Top_floor_v1 (Autodesk Fusion 360 design; units mm, degrees)
Autodesk Fusion 360 part; units mm, degrees
note: some values were not read from the file. Set by a fixed rule: which sketch regions a step uses.
other "Esquisse1"
sketch "Esquisse1" plane through (0, 0, 0) normal (0, 0, 1) x (1, 0, 0) in component "Component"
  line L0 (159, 101.837) -> (-151, 101.837)
  arc A0 (-151, 101.837) -> (-156, 96.837) centre (-151, 96.837) ccw
  line L1 (-156, 96.837) -> (-156, -18.163)
  line L2 (164, -123.163) -> (164, 96.837)
  arc A1 (164, 96.837) -> (159, 101.837) centre (159, 96.837) ccw
  arc A2 (159, -128.163) -> (164, -123.163) centre (159, -123.163) ccw
  line L3 (-26, -128.163) -> (159, -128.163)
  circle A3 centre (155, 92.837) radius 2.75
  circle A4 centre (-147, 92.837) radius 2.75
  circle A5 centre (155, -119.163) radius 2.75
  line L4 (-26, -128.163) -> (-151, -128.163)
  line L5 (-156, -123.163) -> (-156, -18.163)
  arc A6 (-156, -123.163) -> (-151, -128.163) centre (-151, -123.163) ccw
  circle A7 centre (-147, -119.163) radius 2.75
  point P0 (155, 92.837)
  point P1 (-147, 92.837)
  point P2 (155, -119.163)
  dimension "d5" = 5
  dimension "d6" = 5
  dimension "d7" = 5.5
  dimension "d8" = 5.5
  dimension "d9" = 9
  dimension "d10" = 9
  dimension "d11" = 9
  dimension "d12" = 9
  constraint coincident L3.start L4.start
  constraint perpendicular L1 L4
  constraint coincident L1.end L5.end
  constraint perpendicular L3 L5
  constraint tangent L4 A6
  constraint tangent L5 A6
  measures "d5" radius of A6
  measures "d6" radius of A2
  measures "d7" diameter of A7
  measures "d8" diameter of A3
  measures "d9" distance of L2 P0
  measures "d10" distance of L0 P0
  measures "d11" distance of L4 A7.centre
  measures "d12" distance of L5 A7.centre
extrude "Extrusion1" add sketch "Esquisse1" along normal blind 3 in component "Component"
component "Component" placed x (1, 0, 0) y (0, 1, 0) z (0, 0, 1) at (0, 0, 0)
equation "d5 = d6"
equation "d7 = d8"
equation "d11 = d9"
equation "d12 = d10"
